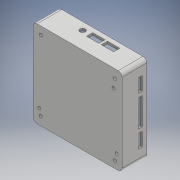
# Autodesk Inventor part: nuc_case_bottom
Saved by Autodesk Inventor 2018 (Build 220112000, 112)
## iProperties
Created: 2017-11-17
Part Number: nuc_case_bottom
Material: Genérico
Document SubType Name: Modeling
Designer: se_ma
Density: 1 g/cm^3
Appearance: Valor por defecto
Author: se_ma
Autodesk Inventor part; units mm, degrees
ref_plane "YZ Plane" through (0, 0, 0) normal (1, 0, 0) x (0, 1, 0)
ref_plane "XZ Plane" through (0, 0, 0) normal (0, 1, 0) x (-1, 0, 0)
ref_plane "XY Plane" through (0, 0, 0) normal (0, 0, 1) x (1, 0, 0)
sketch "Boceto1" plane through (0, 0, 0) normal (0, 1, 0) x (-1, 0, 0)
  line L0 (5, 0) -> (110, 0)
  line L1 (115, -5) -> (115, -107)
  line L2 (110, -112) -> (5, -112)
  line L3 (0, -107) -> (0, -5)
  arc A0 (115, -5) -> (110, 0) centre (110, -5) ccw
  arc A1 (0, -107) -> (5, -112) centre (5, -107) ccw
  arc A2 (110, -112) -> (115, -107) centre (110, -107) ccw
  arc A3 (5, 0) -> (0, -5) centre (5, -5) ccw
  point P0 (0, 0)
  point P1 (115, -112)
  point P2 (115, 0)
  point P3 (0, -112)
  dimension "d0" = 115
  dimension "d1" = 112
  dimension "d2" = 5
  dimension "d3" = 5
  constraints: 8 end point, 8 point on circle, 8 point on line, 8 tangent, 4 centre point, 2 equal radius, 2 parallel, 1 horizontal, 1 perpendicular
  measures "d0" distance of point (115, -112) point (0, -112)
  measures "d1" distance of point (115, 0) point (115, -112)
  measures "d2" radius of A0
  measures "d3" radius of A2
extrude "Extrusión1" add sketch "Boceto1" along normal blind 4
sketch "Boceto2" plane through (0, 4, 0) normal (0, 1, 0) x (1, 0, 0)
  line L0 (-5, 0) -> (-110, 0)
  line L1 (-115, 5) -> (-115, 107)
  line L2 (-110, 112) -> (-5, 112)
  line L3 (0, 107) -> (0, 5)
  arc A0 (-110, 112) -> (-115, 107) centre (-110, 107) ccw
  arc A1 (0, 107) -> (-5, 112) centre (-5, 107) ccw
  arc A2 (-5, 0) -> (0, 5) centre (-5, 5) ccw
  arc A3 (-115, 5) -> (-110, 0) centre (-110, 5) ccw
  line L4 (-110, 0) -> (-5, 0) projected
  line L5 (-5, 112) -> (-110, 112) projected
  line L6 (-115, 107) -> (-115, 5) projected
  line L7 (0, 5) -> (0, 107) projected
  line L8 (-112, 56) -> (-112, 104)
  line L9 (-3, 56) -> (-3, 104)
  line L10 (-107, 109) -> (-8, 109)
  line L11 (-57.5, 3) -> (-8, 3)
  line L12 (-57.5, 3) -> (-107, 3)
  line L13 (-112, 56) -> (-112, 8)
  line L14 (-3, 56) -> (-3, 8)
  arc A4 (-107, 109) -> (-112, 104) centre (-107, 104) ccw
  arc A5 (-3, 104) -> (-8, 109) centre (-8, 104) ccw
  arc A6 (-112, 8) -> (-107, 3) centre (-107, 8) ccw
  arc A7 (-8, 3) -> (-3, 8) centre (-8, 8) ccw
  point P0 (0, 0)
  point P1 (-112, 3)
  constraints: 22 end point, 16 point on circle, 16 tangent, 8 centre point, 6 equal radius, 5 point on line, 3 perpendicular, 2 parallel, 1 horizontal, 1 vertical
extrude "Extrusión2" add sketch "Boceto2" along normal blind 28
sketch "Boceto3" plane through (-110, 0, 0) normal (0, 0, 1) x (1, 0, 0)
  line L0 (110, 0) -> (110, 32) projected
  line L1 (0, 32) -> (105, 32) projected
  line L2 (0, 0) -> (105, 0) projected
  line L3 (46, 26) -> (62, 26)
  line L4 (62, 26) -> (62, 18)
  line L5 (62, 18) -> (46, 18)
  line L6 (46, 18) -> (46, 26)
  line L7 (65, 26) -> (65, 18)
  line L8 (65, 18) -> (81, 18)
  line L9 (81, 18) -> (81, 26)
  line L10 (81, 26) -> (65, 26)
  dimension "d18" = 3
  dimension "d19" = 16
  constraints: 16 end point, 6 perpendicular, 1 horizontal
  measures "d18" distance of L3.end L7.start
  measures "d19" distance of L7.end L8.end
extrude "Extrusión3" cut sketch "Boceto3" against normal blind 3
sketch "Boceto4" plane through (0, 0, -5) normal (1, 0, 0) x (0, 0, -1)
  line L0 (0, 32) -> (102, 32) projected
  line L1 (51, 32) -> (51, 26)
  line L2 (91, 26) -> (91, 21)
  line L3 (11, 21) -> (11, 26)
  line L4 (28.5, 26) -> (28.5, 21)
  line L5 (33.5, 26) -> (33.5, 21)
  line L6 (51, 26) -> (33.5, 26)
  line L7 (11, 26) -> (28.5, 26)
  line L8 (68.5, 26) -> (68.5, 21)
  line L9 (73.5, 26) -> (73.5, 21)
  line L10 (68.5, 26) -> (51, 26)
  line L11 (73.5, 26) -> (91, 26)
  line L12 (73.5, 21) -> (91, 21)
  line L13 (11, 21) -> (28.5, 21)
  line L14 (33.5, 21) -> (68.5, 21)
  point P0 (-5, 0)
  dimension "d22" = 6
  dimension "d23" = 40
  dimension "d24" = 40
  dimension "d25" = 5
  constraints: 28 end point, 3 collinear, 2 horizontal, 1 midpoint, 1 parallel, 1 vertical
  measures "d22" distance of L1.start L1.end
  measures "d23" distance of L1.end L3.end
  measures "d24" distance of L1.end L2.start
  measures "d25" distance of L2.start L2.end
extrude "Extrusión4" cut sketch "Boceto4" against normal blind 115
sketch "Boceto5" plane through (-110, 0, 0) normal (0, 0, 1) x (1, 0, 0)
  line L0 (46, 18) -> (46, 26) projected
  circle A0 centre (37, 22) radius 3.5
  point P0 (110, 0)
  dimension "d35" = 7
  constraints: 1 centre point
  measures "d35" diameter of A0
extrude "Extrusión5" cut sketch "Boceto5" against normal blind 3
sketch "Boceto6" plane through (-5, 0, -112) normal (0, 0, -1) x (-1, 0, 0)
  line L0 (110, 0) -> (110, 32) projected
  line L1 (3, 32) -> (102, 32) projected
  line L2 (8, 25) -> (24, 25)
  line L3 (24, 25) -> (24, 15)
  line L4 (24, 15) -> (8, 15)
  line L5 (8, 15) -> (8, 25)
  line L6 (105, 0) -> (0, 0) projected
  line L7 (28, 32) -> (31, 32) construction
  line L8 (28, 29) -> (42, 29)
  line L9 (42, 29) -> (42, 23)
  line L10 (42, 23) -> (28, 23)
  line L11 (28, 29) -> (28, 23)
  line L12 (28, 23) -> (30, 23) construction
  line L13 (28, 20) -> (42, 20)
  line L14 (42, 20) -> (42, 14)
  line L15 (42, 14) -> (28, 14)
  line L16 (28, 14) -> (28, 20)
  line L17 (49, 25) -> (54, 25)
  line L18 (49, 25) -> (49, 15)
  line L19 (49, 15) -> (64, 15)
  line L20 (64, 15) -> (64, 25)
  line L21 (64, 25) -> (59, 25)
  line L22 (59, 25) -> (59, 26)
  line L23 (59, 26) -> (54, 26)
  line L24 (54, 25) -> (54, 26)
  line L25 (24, 12) -> (79, 12)
  line L26 (79, 12) -> (79, 5)
  line L27 (79, 5) -> (24, 5)
  line L28 (24, 5) -> (24, 12)
  line L29 (64, 25) -> (64, 24)
  arc A0 (87, 24) -> (94, 24) centre (90.5, 24) ccw
  line L30 (87, 24) -> (87, 32)
  line L31 (94, 24) -> (94, 32)
  point P0 (-5, 0)
  dimension "d40" = 16
  dimension "d44" = 3
  dimension "d46" = 14
  dimension "d47" = 6
  dimension "d51" = 6
  dimension "d54" = 5
  dimension "d56" = 10
  dimension "d58" = 15
  dimension "d59" = 3
  dimension "d60" = 55
  dimension "d61" = 7
  dimension "d62" = 1
  dimension "d64" = 7
  constraints: 58 end point, 14 perpendicular, 4 point on line, 3 horizontal, 3 vertical, 2 point on circle, 1 centre point, 1 tangent
  measures "d40" distance of L2.start L2.end
  measures "d44" distance of L7.start L8.start
  measures "d46" distance of L8.start L8.end
  measures "d47" distance of L8.end L9.end
  measures "d51" distance of L13.end L14.end
  measures "d54" distance of L17.start L17.end
  measures "d56" distance of L17.start L18.end
  measures "d58" distance of L18.end L19.end
  measures "d59" distance of L3.end L25.start
  measures "d60" distance of L25.start L25.end
  measures "d61" distance of L25.end L26.end
  measures "d62" distance of L20.end L29.end
  measures "d64" diameter of A0
extrude "Extrusión6" cut sketch "Boceto6" against normal blind 3
sketch "Boceto7" plane through (0, 4, 0) normal (0, 1, 0) x (1, 0, 0)
  line L0 (-3, 104) -> (-3, 8)
  line L1 (-112, 8) -> (-112, 104)
  arc A0 (-107, 109) -> (-112, 104) centre (-107, 104) ccw
  arc A1 (-3, 104) -> (-8, 109) centre (-8, 104) ccw
  arc A2 (-8, 3) -> (-3, 8) centre (-8, 8) ccw
  arc A3 (-112, 8) -> (-107, 3) centre (-107, 8) ccw
  line L2 (-112, 104) -> (-112, 8) projected
  line L3 (-3, 8) -> (-3, 104) projected
  line L4 (-87, 56) -> (-87, 109)
  line L5 (-28, 56) -> (-28, 109)
  line L6 (-87, 109) -> (-87, 34)
  line L7 (-64, 3) -> (-48, 3) projected
  line L8 (-28, 56) -> (-28, 34)
  line L9 (-107, 3) -> (-71, 3)
  line L10 (-41, 3) -> (-8, 3)
  line L11 (-107, 109) -> (-87, 109)
  line L12 (-28, 109) -> (-8, 109)
  line L13 (-56, 8) -> (-36.2245, 8)
  line L14 (-56, 8) -> (-77.303, 8)
  line L15 (-71, 3) -> (-41, 3)
  line L16 (-107, 3) -> (-8, 3) projected
  arc A4 (-87, 34) -> (-77.303, 8) centre (-52.0449, 32.2286) ccw
  arc A5 (-36.2245, 8) -> (-28, 34) centre (-62.8462, 30.7219) ccw
  point P0 (0, 0)
  point P1 (-28, 3)
  dimension "d70" = 75
  dimension "d73" = 35
  dimension "d74" = 35
  constraints: 26 end point, 12 point on circle, 6 centre point, 4 tangent, 3 equal radius, 2 horizontal, 1 collinear, 1 parallel, 1 vertical
  measures "d70" distance of L4.end L6.end
  measures "d73" radius of A4
  measures "d74" radius of A5
extrude "Extrusión7" add sketch "Boceto7" along normal blind 5
fillet "Empalme1" radius 2.5 10 edges at (-87, 4, -71.5) (-87, 9, -71.5) (-28, 4, -71.5) (-28, 9, -71.5) (-29.4759, 4, -20.1661) (-29.4759, 9, -20.1661) (-56.7637, 9, -8) (-56.7637, 4, -8) (-84.8383, 9, -19.9979) (-84.8383, 4, -19.9979)
sketch "Boceto8" plane through (0, 9, 0) normal (0, 1, 0) x (1, 0, 0)
  circle A0 centre (-9, 11) radius 2
  line L0 (0, 112) -> (-9, 112)
  line L1 (-5, 112) -> (-110, 112) projected
  line L2 (-9, 112) -> (-9, 103)
  circle A1 centre (-9, 103) radius 2
  line L3 (0, 112) -> (-7, 112)
  line L4 (-7, 112) -> (-7, 94)
  circle A2 centre (-7, 94) radius 2
  line L5 (-115, 0) -> (-105, 0)
  line L6 (-110, 0) -> (-5, 0) projected
  line L7 (-105, 0) -> (-105, 10)
  circle A3 centre (-105, 10) radius 2
  line L8 (0, 0) -> (-11, 0)
  line L9 (-11, 0) -> (-11, 22.5)
  circle A4 centre (-11, 22.5) radius 2
  line L10 (-115, 112) -> (-105, 112)
  line L11 (-105, 112) -> (-105, 101)
  line L12 (-115, 112) -> (-107, 112)
  line L13 (-107, 112) -> (-107, 93)
  circle A5 centre (-107, 93) radius 2
  circle A6 centre (-105, 101) radius 2
  dimension "d79" = 4
  dimension "d80" = 9
  dimension "d81" = 4
  dimension "d82" = 7
  dimension "d83" = 18
  dimension "d84" = 10
  dimension "d85" = 10
  dimension "d86" = 4
  dimension "d87" = 22.5
  dimension "d88" = 4
  dimension "d89" = 10
  dimension "d90" = 11
  dimension "d91" = 8
  dimension "d92" = 19
  dimension "d93" = 4
  constraints: 24 end point, 7 centre point, 7 point on line, 6 coincident, 6 perpendicular, 1 tangent
  measures "d79" diameter of A0
  measures "d80" distance of L0.end L2.end
  measures "d81" diameter of A1
  measures "d82" distance of L0.start L3.end
  measures "d83" distance of L3.end L4.end
  measures "d84" distance of L5.start L5.end
  measures "d85" distance of L5.end L7.end
  measures "d86" diameter of A3
  measures "d87" distance of L8.end L9.end
  measures "d88" diameter of A4
  measures "d89" distance of L10.start L10.end
  measures "d90" distance of L10.end L11.end
  measures "d91" distance of L10.start L12.end
  measures "d92" distance of L12.end L13.end
  measures "d93" diameter of A5
extrude "Extrusión8" cut sketch "Boceto8" against normal blind 9 contours A0 | A1 | A6 | A2 | A3 | A4 | A5
